Autodesk Fusion 360 part; units mm, degrees
(part 2 of 6)
  line L301 (104.1498, 9.6625) -> (103.164, 16.625)
  line L302 (105.0914, 15.125) -> (104.879, 16.625)
  line L303 (110.8723, 16.625) -> (111.8583, 9.6615)
  line L304 (105.0974, 9.5752) -> (105.8357, 8.8126)
  line L305 (104.679, 16.625) -> (105.5728, 10.3124)
  line L306 (110.938, 9.5499) -> (110.1997, 10.3126)
  line L307 (110.2123, 10.5871) -> (109.3574, 16.625)
  line L308 (104.879, 16.625) -> (109.1574, 16.625)
  line L309 (110.1997, 10.3126) -> (105.8609, 10.3126)
  line L310 (109.3574, 16.625) -> (110.8723, 16.625)
  line L311 (105.5728, 10.3124) -> (104.8998, 9.6625)
  line L312 (122.0778, 15.125) -> (117.7994, 15.125)
  line L313 (117.387, 16.625) -> (115.872, 16.625)
  arc A45 (125.0045, 2.5) -> (125.4996, 3.0701) centre (125.0045, 3) ccw
  circle A46 centre (115.872, 3.375) radius 0.875
  line L314 (117.6362, 9.4625) -> (118.5322, 8.5369)
  line L315 (124.0803, 2.5) -> (125.5803, 2.5)
  line L316 (123.6659, 4) -> (119.3766, 4)
  line L317 (118.5689, 10.3126) -> (117.8054, 9.5752)
  line L318 (119.387, 2.5) -> (117.872, 2.5)
  line L319 (117.872, 2.5) -> (116.8862, 9.4625)
  line L320 (123.1846, 8.8263) -> (124.0803, 2.5)
  line L321 (123.8783, 2.5) -> (123.6659, 4)
  line L322 (122.8824, 8.8126) -> (123.646, 9.5499)
  line L323 (124.5663, 9.6615) -> (123.8163, 9.6615)
  line L324 (125.5803, 2.5) -> (124.5944, 9.4635)
  arc A47 (116.4478, 16.625) -> (115.9527, 16.0549) centre (116.4478, 16.125) ccw
  line L325 (119.589, 2.5) -> (123.8783, 2.5)
  line L326 (118.5322, 8.5369) -> (119.387, 2.5)
  line L327 (123.8444, 9.4635) -> (123.1846, 8.8263)
  line L328 (119.3766, 4) -> (119.589, 2.5)
  line L329 (118.5437, 8.8126) -> (122.8824, 8.8126)
  line L330 (123.8163, 9.6615) -> (122.9203, 10.5871)
  line L331 (116.8862, 9.4625) -> (117.6362, 9.4625)
  line L332 (124.5944, 9.4635) -> (123.8444, 9.4635)
  arc A48 (117.8111, 2.9299) -> (118.3062, 2.5) centre (118.3062, 3) ccw
  line L333 (117.6078, 9.6625) -> (116.8578, 9.6625)
  line L334 (121.8654, 16.625) -> (122.0778, 15.125)
  arc A49 (123.6412, 16.1951) -> (123.1461, 16.625) centre (123.1461, 16.125) ccw
  line L335 (116.8578, 9.6625) -> (115.872, 16.625)
  line L336 (117.7994, 15.125) -> (117.587, 16.625)
  line L337 (123.5803, 16.625) -> (124.5663, 9.6615)
  line L338 (117.8054, 9.5752) -> (118.5437, 8.8126)
  line L339 (117.387, 16.625) -> (118.2808, 10.3124)
  line L340 (123.646, 9.5499) -> (122.9077, 10.3126)
  line L341 (122.9203, 10.5871) -> (122.0654, 16.625)
  line L342 (117.587, 16.625) -> (121.8654, 16.625)
  line L343 (122.9077, 10.3126) -> (118.5689, 10.3126)
  line L344 (122.0654, 16.625) -> (123.5803, 16.625)
  line L345 (118.2808, 10.3124) -> (117.6078, 9.6625)
  line L346 (134.7858, 15.125) -> (130.5074, 15.125)
  line L347 (130.095, 16.625) -> (128.58, 16.625)
  arc A50 (137.7125, 2.5) -> (138.2076, 3.0701) centre (137.7125, 3) ccw
  circle A51 centre (128.58, 3.375) radius 0.875
  line L348 (130.3442, 9.4625) -> (131.2402, 8.5369)
  line L349 (136.7883, 2.5) -> (138.2883, 2.5)
  line L350 (136.3739, 4) -> (132.0846, 4)
  line L351 (131.2769, 10.3126) -> (130.5134, 9.5752)
  line L352 (132.095, 2.5) -> (130.58, 2.5)
  line L353 (130.58, 2.5) -> (129.5942, 9.4625)
  line L354 (135.8926, 8.8263) -> (136.7883, 2.5)
  line L355 (136.5863, 2.5) -> (136.3739, 4)
  line L356 (135.5904, 8.8126) -> (136.354, 9.5499)
  line L357 (137.2743, 9.6615) -> (136.5243, 9.6615)
  line L358 (138.2883, 2.5) -> (137.3024, 9.4635)
  arc A52 (129.1558, 16.625) -> (128.6607, 16.0549) centre (129.1558, 16.125) ccw
  line L359 (132.297, 2.5) -> (136.5863, 2.5)
  line L360 (131.2402, 8.5369) -> (132.095, 2.5)
  line L361 (136.5524, 9.4635) -> (135.8926, 8.8263)
  line L362 (132.0846, 4) -> (132.297, 2.5)
  line L363 (131.2517, 8.8126) -> (135.5904, 8.8126)
  line L364 (136.5243, 9.6615) -> (135.6283, 10.5871)
  line L365 (129.5942, 9.4625) -> (130.3442, 9.4625)
  line L366 (137.3024, 9.4635) -> (136.5524, 9.4635)
  arc A53 (130.5191, 2.9299) -> (131.0142, 2.5) centre (131.0142, 3) ccw
  line L367 (130.3158, 9.6625) -> (129.5658, 9.6625)
  line L368 (134.5734, 16.625) -> (134.7858, 15.125)
  arc A54 (136.3492, 16.1951) -> (135.8541, 16.625) centre (135.8541, 16.125) ccw
  line L369 (129.5658, 9.6625) -> (128.58, 16.625)
  line L370 (130.5074, 15.125) -> (130.295, 16.625)
  line L371 (136.2883, 16.625) -> (137.2743, 9.6615)
  line L372 (130.5134, 9.5752) -> (131.2517, 8.8126)
  line L373 (130.095, 16.625) -> (130.9888, 10.3124)
  line L374 (136.354, 9.5499) -> (135.6157, 10.3126)
  line L375 (135.6283, 10.5871) -> (134.7734, 16.625)
  line L376 (130.295, 16.625) -> (134.5734, 16.625)
  line L377 (135.6157, 10.3126) -> (131.2769, 10.3126)
  line L378 (134.7734, 16.625) -> (136.2883, 16.625)
  line L379 (130.9888, 10.3124) -> (130.3158, 9.6625)
  line L380 (147.4938, 15.125) -> (143.2154, 15.125)
  line L381 (142.803, 16.625) -> (141.288, 16.625)
  arc A55 (150.4205, 2.5) -> (150.9156, 3.0701) centre (150.4205, 3) ccw
  circle A56 centre (141.288, 3.375) radius 0.875
  line L382 (143.0522, 9.4625) -> (143.9482, 8.5369)
  line L383 (149.4963, 2.5) -> (150.9963, 2.5)
  line L384 (149.0819, 4) -> (144.7926, 4)
  line L385 (143.9849, 10.3126) -> (143.2214, 9.5752)
  line L386 (144.803, 2.5) -> (143.288, 2.5)
  line L387 (143.288, 2.5) -> (142.3022, 9.4625)
  line L388 (148.6006, 8.8263) -> (149.4963, 2.5)
  line L389 (149.2943, 2.5) -> (149.0819, 4)
  line L390 (148.2984, 8.8126) -> (149.062, 9.5499)
  line L391 (149.9823, 9.6615) -> (149.2323, 9.6615)
  line L392 (150.9963, 2.5) -> (150.0104, 9.4635)
  arc A57 (141.8638, 16.625) -> (141.3687, 16.0549) centre (141.8638, 16.125) ccw
  line L393 (145.005, 2.5) -> (149.2943, 2.5)
  line L394 (143.9482, 8.5369) -> (144.803, 2.5)
  line L395 (149.2604, 9.4635) -> (148.6006, 8.8263)
  line L396 (144.7926, 4) -> (145.005, 2.5)
  line L397 (143.9597, 8.8126) -> (148.2984, 8.8126)
  line L398 (149.2323, 9.6615) -> (148.3363, 10.5871)
  line L399 (142.3022, 9.4625) -> (143.0522, 9.4625)
  line L400 (150.0104, 9.4635) -> (149.2604, 9.4635)
  arc A58 (143.2271, 2.9299) -> (143.7222, 2.5) centre (143.7222, 3) ccw
  line L401 (143.0238, 9.6625) -> (142.2738, 9.6625)
  line L402 (147.2814, 16.625) -> (147.4938, 15.125)
  arc A59 (149.0572, 16.1951) -> (148.5621, 16.625) centre (148.5621, 16.125) ccw
  line L403 (142.2738, 9.6625) -> (141.288, 16.625)
  line L404 (143.2154, 15.125) -> (143.003, 16.625)
  line L405 (148.9963, 16.625) -> (149.9823, 9.6615)
  line L406 (143.2214, 9.5752) -> (143.9597, 8.8126)
  line L407 (142.803, 16.625) -> (143.6968, 10.3124)
  line L408 (149.062, 9.5499) -> (148.3237, 10.3126)
  line L409 (148.3363, 10.5871) -> (147.4814, 16.625)
  line L410 (143.003, 16.625) -> (147.2814, 16.625)
  line L411 (148.3237, 10.3126) -> (143.9849, 10.3126)
  line L412 (147.4814, 16.625) -> (148.9963, 16.625)
  line L413 (143.6968, 10.3124) -> (143.0238, 9.6625)
  line L414 (160.2018, 15.125) -> (155.9234, 15.125)
  line L415 (155.511, 16.625) -> (153.996, 16.625)
  arc A60 (163.1285, 2.5) -> (163.6236, 3.0701) centre (163.1285, 3) ccw
  circle A61 centre (153.996, 3.375) radius 0.875
  line L416 (155.7602, 9.4625) -> (156.6562, 8.5369)
  line L417 (162.2043, 2.5) -> (163.7043, 2.5)
  line L418 (161.7899, 4) -> (157.5006, 4)
  line L419 (156.6929, 10.3126) -> (155.9294, 9.5752)
  line L420 (157.511, 2.5) -> (155.996, 2.5)
  line L421 (155.996, 2.5) -> (155.0102, 9.4625)
  line L422 (161.3086, 8.8263) -> (162.2043, 2.5)
  line L423 (162.0023, 2.5) -> (161.7899, 4)
  line L424 (161.0064, 8.8126) -> (161.77, 9.5499)
  line L425 (162.6903, 9.6615) -> (161.9403, 9.6615)
  line L426 (163.7043, 2.5) -> (162.7184, 9.4635)
  arc A62 (154.5718, 16.625) -> (154.0767, 16.0549) centre (154.5718, 16.125) ccw
  line L427 (157.713, 2.5) -> (162.0023, 2.5)
  line L428 (156.6562, 8.5369) -> (157.511, 2.5)
  line L429 (161.9684, 9.4635) -> (161.3086, 8.8263)
  line L430 (157.5006, 4) -> (157.713, 2.5)
  line L431 (156.6677, 8.8126) -> (161.0064, 8.8126)
  line L432 (161.9403, 9.6615) -> (161.0443, 10.5871)
  line L433 (155.0102, 9.4625) -> (155.7602, 9.4625)
  line L434 (162.7184, 9.4635) -> (161.9684, 9.4635)
  arc A63 (155.9351, 2.9299) -> (156.4302, 2.5) centre (156.4302, 3) ccw
  line L435 (155.7318, 9.6625) -> (154.9818, 9.6625)
  line L436 (159.9894, 16.625) -> (160.2018, 15.125)
  arc A64 (161.7652, 16.1951) -> (161.2701, 16.625) centre (161.2701, 16.125) ccw
  line L437 (154.9818, 9.6625) -> (153.996, 16.625)
  line L438 (155.9234, 15.125) -> (155.711, 16.625)
  line L439 (161.7043, 16.625) -> (162.6903, 9.6615)
  line L440 (155.9294, 9.5752) -> (156.6677, 8.8126)
  line L441 (155.511, 16.625) -> (156.4048, 10.3124)
  line L442 (161.77, 9.5499) -> (161.0317, 10.3126)
  line L443 (161.0443, 10.5871) -> (160.1894, 16.625)
  line L444 (155.711, 16.625) -> (159.9894, 16.625)
  line L445 (161.0317, 10.3126) -> (156.6929, 10.3126)
  line L446 (160.1894, 16.625) -> (161.7043, 16.625)
  line L447 (156.4048, 10.3124) -> (155.7318, 9.6625)
  line L448 (172.9098, 15.125) -> (168.6314, 15.125)
  line L449 (168.219, 16.625) -> (166.704, 16.625)
  arc A65 (175.8365, 2.5) -> (176.3316, 3.0701) centre (175.8365, 3) ccw
  circle A66 centre (166.704, 3.375) radius 0.875
  line L450 (168.4682, 9.4625) -> (169.3642, 8.5369)
  line L451 (174.9123, 2.5) -> (176.4123, 2.5)
  line L452 (174.4979, 4) -> (170.2086, 4)
  line L453 (169.4009, 10.3126) -> (168.6374, 9.5752)
  line L454 (170.219, 2.5) -> (168.704, 2.5)
  line L455 (168.704, 2.5) -> (167.7182, 9.4625)
  line L456 (174.0166, 8.8263) -> (174.9123, 2.5)
  line L457 (174.7103, 2.5) -> (174.4979, 4)
  line L458 (173.7144, 8.8126) -> (174.478, 9.5499)
  line L459 (175.3983, 9.6615) -> (174.6483, 9.6615)
  line L460 (176.4123, 2.5) -> (175.4264, 9.4635)
  arc A67 (167.2798, 16.625) -> (166.7847, 16.0549) centre (167.2798, 16.125) ccw
  line L461 (170.421, 2.5) -> (174.7103, 2.5)
  line L462 (169.3642, 8.5369) -> (170.219, 2.5)
  line L463 (174.6764, 9.4635) -> (174.0166, 8.8263)
  line L464 (170.2086, 4) -> (170.421, 2.5)
  line L465 (169.3757, 8.8126) -> (173.7144, 8.8126)
  line L466 (174.6483, 9.6615) -> (173.7523, 10.5871)
  line L467 (167.7182, 9.4625) -> (168.4682, 9.4625)
  line L468 (175.4264, 9.4635) -> (174.6764, 9.4635)
  arc A68 (168.6431, 2.9299) -> (169.1382, 2.5) centre (169.1382, 3) ccw
  line L469 (168.4398, 9.6625) -> (167.6898, 9.6625)
  line L470 (172.6974, 16.625) -> (172.9098, 15.125)
  arc A69 (174.4732, 16.1951) -> (173.9781, 16.625) centre (173.9781, 16.125) ccw
  line L471 (167.6898, 9.6625) -> (166.704, 16.625)
  line L472 (168.6314, 15.125) -> (168.419, 16.625)
  line L473 (174.4123, 16.625) -> (175.3983, 9.6615)
  line L474 (168.6374, 9.5752) -> (169.3757, 8.8126)
  line L475 (168.219, 16.625) -> (169.1128, 10.3124)
  line L476 (174.478, 9.5499) -> (173.7397, 10.3126)
  line L477 (173.7523, 10.5871) -> (172.8974, 16.625)
  line L478 (168.419, 16.625) -> (172.6974, 16.625)
  line L479 (173.7397, 10.3126) -> (169.4009, 10.3126)
  line L480 (172.8974, 16.625) -> (174.4123, 16.625)
  line L481 (169.1128, 10.3124) -> (168.4398, 9.6625)
  line L482 (185.6178, 15.125) -> (181.3394, 15.125)
  line L483 (180.927, 16.625) -> (179.412, 16.625)
  arc A70 (188.5445, 2.5) -> (189.0396, 3.0701) centre (188.5445, 3) ccw
  circle A71 centre (179.412, 3.375) radius 0.875
  line L484 (181.1762, 9.4625) -> (182.0722, 8.5369)
  line L485 (187.6203, 2.5) -> (189.1203, 2.5)
  line L486 (187.2059, 4) -> (182.9166, 4)
  line L487 (182.1089, 10.3126) -> (181.3454, 9.5752)
  line L488 (182.927, 2.5) -> (181.412, 2.5)
  line L489 (181.412, 2.5) -> (180.4262, 9.4625)
  line L490 (186.7246, 8.8263) -> (187.6203, 2.5)
  line L491 (187.4183, 2.5) -> (187.2059, 4)
  line L492 (186.4224, 8.8126) -> (187.186, 9.5499)
  line L493 (188.1063, 9.6615) -> (187.3563, 9.6615)
  line L494 (189.1203, 2.5) -> (188.1344, 9.4635)
  arc A72 (179.9878, 16.625) -> (179.4927, 16.0549) centre (179.9878, 16.125) ccw
  line L495 (183.129, 2.5) -> (187.4183, 2.5)
  line L496 (182.0722, 8.5369) -> (182.927, 2.5)
  line L497 (187.3844, 9.4635) -> (186.7246, 8.8263)
  line L498 (182.9166, 4) -> (183.129, 2.5)
  line L499 (182.0837, 8.8126) -> (186.4224, 8.8126)
  line L500 (187.3563, 9.6615) -> (186.4603, 10.5871)
  line L501 (180.4262, 9.4625) -> (181.1762, 9.4625)
  line L502 (188.1344, 9.4635) -> (187.3844, 9.4635)
  arc A73 (181.3511, 2.9299) -> (181.8462, 2.5) centre (181.8462, 3) ccw
  line L503 (181.1478, 9.6625) -> (180.3978, 9.6625)
  line L504 (185.4054, 16.625) -> (185.6178, 15.125)
  arc A74 (187.1812, 16.1951) -> (186.6861, 16.625) centre (186.6861, 16.125) ccw
  line L505 (180.3978, 9.6625) -> (179.412, 16.625)
  line L506 (181.3394, 15.125) -> (181.127, 16.625)
  line L507 (187.1203, 16.625) -> (188.1063, 9.6615)
  line L508 (181.3454, 9.5752) -> (182.0837, 8.8126)
  line L509 (180.927, 16.625) -> (181.8208, 10.3124)
  line L510 (187.186, 9.5499) -> (186.4477, 10.3126)
  line L511 (186.4603, 10.5871) -> (185.6054, 16.625)
  line L512 (181.127, 16.625) -> (185.4054, 16.625)
  line L513 (186.4477, 10.3126) -> (182.1089, 10.3126)
  line L514 (185.6054, 16.625) -> (187.1203, 16.625)
  line L515 (181.8208, 10.3124) -> (181.1478, 9.6625)
  line L516 (198.3258, 15.125) -> (194.0474, 15.125)
  line L517 (193.635, 16.625) -> (192.12, 16.625)
  arc A75 (201.2525, 2.5) -> (201.7476, 3.0701) centre (201.2525, 3) ccw
  circle A76 centre (192.12, 3.375) radius 0.875
  line L518 (193.8842, 9.4625) -> (194.7802, 8.5369)
  line L519 (200.3283, 2.5) -> (201.8283, 2.5)
  line L520 (199.9139, 4) -> (195.6246, 4)
  line L521 (194.8169, 10.3126) -> (194.0534, 9.5752)
  line L522 (195.635, 2.5) -> (194.12, 2.5)
  line L523 (194.12, 2.5) -> (193.1342, 9.4625)
  line L524 (199.4326, 8.8263) -> (200.3283, 2.5)
  line L525 (200.1263, 2.5) -> (199.9139, 4)
  line L526 (199.1304, 8.8126) -> (199.894, 9.5499)
  line L527 (200.8143, 9.6615) -> (200.0643, 9.6615)
  line L528 (201.8283, 2.5) -> (200.8424, 9.4635)
  arc A77 (192.6958, 16.625) -> (192.2007, 16.0549) centre (192.6958, 16.125) ccw
  line L529 (195.837, 2.5) -> (200.1263, 2.5)
  line L530 (194.7802, 8.5369) -> (195.635, 2.5)
  line L531 (200.0924, 9.4635) -> (199.4326, 8.8263)
  line L532 (195.6246, 4) -> (195.837, 2.5)
  line L533 (194.7917, 8.8126) -> (199.1304, 8.8126)
  line L534 (200.0643, 9.6615) -> (199.1683, 10.5871)
  line L535 (193.1342, 9.4625) -> (193.8842, 9.4625)
  line L536 (200.8424, 9.4635) -> (200.0924, 9.4635)
  arc A78 (194.0591, 2.9299) -> (194.5542, 2.5) centre (194.5542, 3) ccw
  line L537 (193.8558, 9.6625) -> (193.1058, 9.6625)
  line L538 (198.1134, 16.625) -> (198.3258, 15.125)
  arc A79 (199.8892, 16.1951) -> (199.3941, 16.625) centre (199.3941, 16.125) ccw
  line L539 (193.1058, 9.6625) -> (192.12, 16.625)
  line L540 (194.0474, 15.125) -> (193.835, 16.625)
  line L541 (199.8283, 16.625) -> (200.8143, 9.6615)
  line L542 (194.0534, 9.5752) -> (194.7917, 8.8126)
  line L543 (193.635, 16.625) -> (194.5288, 10.3124)
  line L544 (199.894, 9.5499) -> (199.1557, 10.3126)
  line L545 (199.1683, 10.5871) -> (198.3134, 16.625)
  line L546 (193.835, 16.625) -> (198.1134, 16.625)
  line L547 (199.1557, 10.3126) -> (194.8169, 10.3126)
  line L548 (198.3134, 16.625) -> (199.8283, 16.625)
  line L549 (194.5288, 10.3124) -> (193.8558, 9.6625)
  line L550 (7.7058, 34.25) -> (3.4274, 34.25)
  line L551 (3.015, 35.75) -> (1.5, 35.75)
  arc A80 (10.6325, 21.625) -> (11.1276, 22.1951) centre (10.6325, 22.125) ccw
  circle A81 centre (1.5, 22.5) radius 0.875
  line L552 (3.2642, 28.5875) -> (4.1602, 27.6619)
  line L553 (9.7083, 21.625) -> (11.2083, 21.625)
  line L554 (9.2939, 23.125) -> (5.0046, 23.125)
  line L555 (4.1969, 29.4376) -> (3.4334, 28.7002)
  line L556 (5.015, 21.625) -> (3.5, 21.625)
  line L557 (3.5, 21.625) -> (2.5142, 28.5875)
  line L558 (8.8126, 27.9513) -> (9.7083, 21.625)
  line L559 (9.5063, 21.625) -> (9.2939, 23.125)
  line L560 (8.5104, 27.9376) -> (9.274, 28.6749)
  line L561 (10.1943, 28.7865) -> (9.4443, 28.7865)
  line L562 (11.2083, 21.625) -> (10.2224, 28.5885)
  arc A82 (2.0758, 35.75) -> (1.5807, 35.1799) centre (2.0758, 35.25) ccw
  line L563 (5.217, 21.625) -> (9.5063, 21.625)
  line L564 (4.1602, 27.6619) -> (5.015, 21.625)
  line L565 (9.4724, 28.5885) -> (8.8126, 27.9513)
  line L566 (5.0046, 23.125) -> (5.217, 21.625)
  line L567 (4.1717, 27.9376) -> (8.5104, 27.9376)
  line L568 (9.4443, 28.7865) -> (8.5483, 29.7121)
  line L569 (2.5142, 28.5875) -> (3.2642, 28.5875)
  line L570 (10.2224, 28.5885) -> (9.4724, 28.5885)
  arc A83 (3.4391, 22.0549) -> (3.9342, 21.625) centre (3.9342, 22.125) ccw
  line L571 (3.2358, 28.7875) -> (2.4858, 28.7875)
  line L572 (7.4934, 35.75) -> (7.7058, 34.25)
  arc A84 (9.2692, 35.3201) -> (8.7741, 35.75) centre (8.7741, 35.25) ccw
  line L573 (2.4858, 28.7875) -> (1.5, 35.75)
  line L574 (3.4274, 34.25) -> (3.215, 35.75)
  line L575 (9.2083, 35.75) -> (10.1943, 28.7865)
  line L576 (3.4334, 28.7002) -> (4.1717, 27.9376)
  line L577 (3.015, 35.75) -> (3.9088, 29.4374)
  line L578 (9.274, 28.6749) -> (8.5357, 29.4376)
  line L579 (8.5483, 29.7121) -> (7.6934, 35.75)
  line L580 (3.215, 35.75) -> (7.4934, 35.75)
  line L581 (8.5357, 29.4376) -> (4.1969, 29.4376)
  line L582 (7.6934, 35.75) -> (9.2083, 35.75)
  line L583 (3.9088, 29.4374) -> (3.2358, 28.7875)
  line L584 (20.4138, 34.25) -> (16.1354, 34.25)
  line L585 (15.723, 35.75) -> (14.208, 35.75)
  arc A85 (23.3405, 21.625) -> (23.8356, 22.1951) centre (23.3405, 22.125) ccw
  circle A86 centre (14.208, 22.5) radius 0.875
  line L586 (15.9722, 28.5875) -> (16.8682, 27.6619)
  line L587 (22.4163, 21.625) -> (23.9163, 21.625)
  line L588 (22.0019, 23.125) -> (17.7126, 23.125)
  line L589 (16.9049, 29.4376) -> (16.1414, 28.7002)
  line L590 (17.723, 21.625) -> (16.208, 21.625)
  line L591 (16.208, 21.625) -> (15.2222, 28.5875)
  line L592 (21.5206, 27.9513) -> (22.4163, 21.625)
  line L593 (22.2143, 21.625) -> (22.0019, 23.125)
  line L594 (21.2184, 27.9376) -> (21.982, 28.6749)
  line L595 (22.9023, 28.7865) -> (22.1523, 28.7865)
  line L596 (23.9163, 21.625) -> (22.9304, 28.5885)
  arc A87 (14.7838, 35.75) -> (14.2887, 35.1799) centre (14.7838, 35.25) ccw
  line L597 (17.925, 21.625) -> (22.2143, 21.625)
  line L598 (16.8682, 27.6619) -> (17.723, 21.625)
  line L599 (22.1804, 28.5885) -> (21.5206, 27.9513)
  line L600 (17.7126, 23.125) -> (17.925, 21.625)
  line L601 (16.8797, 27.9376) -> (21.2184, 27.9376)
  line L602 (22.1523, 28.7865) -> (21.2563, 29.7121)
  line L603 (15.2222, 28.5875) -> (15.9722, 28.5875)
  line L604 (22.9304, 28.5885) -> (22.1804, 28.5885)
  arc A88 (16.1471, 22.0549) -> (16.6422, 21.625) centre (16.6422, 22.125) ccw
  line L605 (15.9438, 28.7875) -> (15.1938, 28.7875)
  line L606 (20.2014, 35.75) -> (20.4138, 34.25)
  arc A89 (21.9772, 35.3201) -> (21.4821, 35.75) centre (21.4821, 35.25) ccw
  line L607 (15.1938, 28.7875) -> (14.208, 35.75)
  line L608 (16.1354, 34.25) -> (15.923, 35.75)
  line L609 (21.9163, 35.75) -> (22.9023, 28.7865)
  line L610 (16.1414, 28.7002) -> (16.8797, 27.9376)
  line L611 (15.723, 35.75) -> (16.6168, 29.4374)
  line L612 (21.982, 28.6749) -> (21.2437, 29.4376)
  line L613 (21.2563, 29.7121) -> (20.4014, 35.75)
  line L614 (15.923, 35.75) -> (20.2014, 35.75)
  line L615 (21.2437, 29.4376) -> (16.9049, 29.4376)
  line L616 (20.4014, 35.75) -> (21.9163, 35.75)
  line L617 (16.6168, 29.4374) -> (15.9438, 28.7875)
  line L618 (33.1218, 34.25) -> (28.8434, 34.25)
  line L619 (28.431, 35.75) -> (26.916, 35.75)
  arc A90 (36.0485, 21.625) -> (36.5436, 22.1951) centre (36.0485, 22.125) ccw
  circle A91 centre (26.916, 22.5) radius 0.875
  line L620 (28.6802, 28.5875) -> (29.5762, 27.6619)
  line L621 (35.1243, 21.625) -> (36.6243, 21.625)
  line L622 (34.7099, 23.125) -> (30.4206, 23.125)
  line L623 (29.6129, 29.4376) -> (28.8494, 28.7002)
  line L624 (30.431, 21.625) -> (28.916, 21.625)
  line L625 (28.916, 21.625) -> (27.9302, 28.5875)
  line L626 (34.2286, 27.9513) -> (35.1243, 21.625)
  line L627 (34.9223, 21.625) -> (34.7099, 23.125)
  line L628 (33.9264, 27.9376) -> (34.69, 28.6749)
  line L629 (35.6103, 28.7865) -> (34.8603, 28.7865)
  line L630 (36.6243, 21.625) -> (35.6384, 28.5885)
  arc A92 (27.4918, 35.75) -> (26.9967, 35.1799) centre (27.4918, 35.25) ccw
  line L631 (30.633, 21.625) -> (34.9223, 21.625)
  line L632 (29.5762, 27.6619) -> (30.431, 21.625)
  line L633 (34.8884, 28.5885) -> (34.2286, 27.9513)
  line L634 (30.4206, 23.125) -> (30.633, 21.625)
  line L635 (29.5877, 27.9376) -> (33.9264, 27.9376)
  line L636 (34.8603, 28.7865) -> (33.9643, 29.7121)
  line L637 (27.9302, 28.5875) -> (28.6802, 28.5875)
  line L638 (35.6384, 28.5885) -> (34.8884, 28.5885)
  arc A93 (28.8551, 22.0549) -> (29.3502, 21.625) centre (29.3502, 22.125) ccw
  line L639 (28.6518, 28.7875) -> (27.9018, 28.7875)
  line L640 (32.9094, 35.75) -> (33.1218, 34.25)
  arc A94 (34.6852, 35.3201) -> (34.1901, 35.75) centre (34.1901, 35.25) ccw
  line L641 (27.9018, 28.7875) -> (26.916, 35.75)
  line L642 (28.8434, 34.25) -> (28.631, 35.75)
  line L643 (34.6243, 35.75) -> (35.6103, 28.7865)
  line L644 (28.8494, 28.7002) -> (29.5877, 27.9376)
  line L645 (28.431, 35.75) -> (29.3248, 29.4374)
  line L646 (34.69, 28.6749) -> (33.9517, 29.4376)
  line L647 (33.9643, 29.7121) -> (33.1094, 35.75)
  line L648 (28.631, 35.75) -> (32.9094, 35.75)
  line L649 (33.9517, 29.4376) -> (29.6129, 29.4376)
  line L650 (33.1094, 35.75) -> (34.6243, 35.75)
  line L651 (29.3248, 29.4374) -> (28.6518, 28.7875)
  line L652 (45.8298, 34.25) -> (41.5514, 34.25)
  line L653 (41.139, 35.75) -> (39.624, 35.75)
  arc A95 (48.7565, 21.625) -> (49.2516, 22.1951) centre (48.7565, 22.125) ccw
  circle A96 centre (39.624, 22.5) radius 0.875
  line L654 (41.3882, 28.5875) -> (42.2842, 27.6619)
  line L655 (47.8323, 21.625) -> (49.3323, 21.625)
  line L656 (47.4179, 23.125) -> (43.1286, 23.125)
  line L657 (42.3209, 29.4376) -> (41.5574, 28.7002)
  line L658 (43.139, 21.625) -> (41.624, 21.625)
  line L659 (41.624, 21.625) -> (40.6382, 28.5875)
  line L660 (46.9366, 27.9513) -> (47.8323, 21.625)
  line L661 (47.6303, 21.625) -> (47.4179, 23.125)
  line L662 (46.6344, 27.9376) -> (47.398, 28.6749)
  line L663 (48.3183, 28.7865) -> (47.5683, 28.7865)
  line L664 (49.3323, 21.625) -> (48.3464, 28.5885)
  arc A97 (40.1998, 35.75) -> (39.7047, 35.1799) centre (40.1998, 35.25) ccw
  line L665 (43.341, 21.625) -> (47.6303, 21.625)
  line L666 (42.2842, 27.6619) -> (43.139, 21.625)
  line L667 (47.5964, 28.5885) -> (46.9366, 27.9513)
  line L668 (43.1286, 23.125) -> (43.341, 21.625)
  line L669 (42.2957, 27.9376) -> (46.6344, 27.9376)
  line L670 (47.5683, 28.7865) -> (46.6723, 29.7121)
  line L671 (40.6382, 28.5875) -> (41.3882, 28.5875)
  line L672 (48.3464, 28.5885) -> (47.5964, 28.5885)
  arc A98 (41.5631, 22.0549) -> (42.0582, 21.625) centre (42.0582, 22.125) ccw
  line L673 (41.3598, 28.7875) -> (40.6098, 28.7875)
  line L674 (45.6174, 35.75) -> (45.8298, 34.25)
  arc A99 (47.3932, 35.3201) -> (46.8981, 35.75) centre (46.8981, 35.25) ccw
  line L675 (40.6098, 28.7875) -> (39.624, 35.75)
  line L676 (41.5514, 34.25) -> (41.339, 35.75)
  line L677 (47.3323, 35.75) -> (48.3183, 28.7865)
  line L678 (41.5574, 28.7002) -> (42.2957, 27.9376)
  line L679 (41.139, 35.75) -> (42.0328, 29.4374)
  line L680 (47.398, 28.6749) -> (46.6597, 29.4376)
  line L681 (46.6723, 29.7121) -> (45.8174, 35.75)
  line L682 (41.339, 35.75) -> (45.6174, 35.75)
  line L683 (46.6597, 29.4376) -> (42.3209, 29.4376)
  line L684 (45.8174, 35.75) -> (47.3323, 35.75)
  line L685 (42.0328, 29.4374) -> (41.3598, 28.7875)
  line L686 (58.5378, 34.25) -> (54.2594, 34.25)
  line L687 (53.847, 35.75) -> (52.332, 35.75)
  arc A100 (61.4645, 21.625) -> (61.9596, 22.1951) centre (61.4645, 22.125) ccw
  circle A101 centre (52.332, 22.5) radius 0.875
  line L688 (54.0962, 28.5875) -> (54.9922, 27.6619)
  line L689 (60.5403, 21.625) -> (62.0403, 21.625)
  line L690 (60.1259, 23.125) -> (55.8366, 23.125)
  line L691 (55.0289, 29.4376) -> (54.2654, 28.7002)
  line L692 (55.847, 21.625) -> (54.332, 21.625)
  line L693 (54.332, 21.625) -> (53.3462, 28.5875)
  line L694 (59.6446, 27.9513) -> (60.5403, 21.625)
  line L695 (60.3383, 21.625) -> (60.1259, 23.125)
  line L696 (59.3424, 27.9376) -> (60.106, 28.6749)
  line L697 (61.0263, 28.7865) -> (60.2763, 28.7865)
  line L698 (62.0403, 21.625) -> (61.0544, 28.5885)
  arc A102 (52.9078, 35.75) -> (52.4127, 35.1799) centre (52.9078, 35.25) ccw
  line L699 (56.049, 21.625) -> (60.3383, 21.625)
  line L700 (54.9922, 27.6619) -> (55.847, 21.625)
  line L701 (60.3044, 28.5885) -> (59.6446, 27.9513)
  line L702 (55.8366, 23.125) -> (56.049, 21.625)
  line L703 (55.0037, 27.9376) -> (59.3424, 27.9376)
  line L704 (60.2763, 28.7865) -> (59.3803, 29.7121)
  line L705 (53.3462, 28.5875) -> (54.0962, 28.5875)
  line L706 (61.0544, 28.5885) -> (60.3044, 28.5885)
  arc A103 (54.2711, 22.0549) -> (54.7662, 21.625) centre (54.7662, 22.125) ccw
  line L707 (54.0678, 28.7875) -> (53.3178, 28.7875)
  line L708 (58.3254, 35.75) -> (58.5378, 34.25)
  arc A104 (60.1012, 35.3201) -> (59.6061, 35.75) centre (59.6061, 35.25) ccw
  line L709 (53.3178, 28.7875) -> (52.332, 35.75)
  line L710 (54.2594, 34.25) -> (54.047, 35.75)
  line L711 (60.0403, 35.75) -> (61.0263, 28.7865)
  line L712 (54.2654, 28.7002) -> (55.0037, 27.9376)
  line L713 (53.847, 35.75) -> (54.7408, 29.4374)
  line L714 (60.106, 28.6749) -> (59.3677, 29.4376)
  line L715 (59.3803, 29.7121) -> (58.5254, 35.75)
  line L716 (54.047, 35.75) -> (58.3254, 35.75)
  line L717 (59.3677, 29.4376) -> (55.0289, 29.4376)
  line L718 (58.5254, 35.75) -> (60.0403, 35.75)
  line L719 (54.7408, 29.4374) -> (54.0678, 28.7875)
  line L720 (71.2458, 34.25) -> (66.9674, 34.25)
  line L721 (66.555, 35.75) -> (65.04, 35.75)
  arc A105 (74.1725, 21.625) -> (74.6676, 22.1951) centre (74.1725, 22.125) ccw
  circle A106 centre (65.04, 22.5) radius 0.875
  line L722 (66.8042, 28.5875) -> (67.7002, 27.6619)
  line L723 (73.2483, 21.625) -> (74.7483, 21.625)
  line L724 (72.8339, 23.125) -> (68.5446, 23.125)
  line L725 (67.7369, 29.4376) -> (66.9734, 28.7002)
  line L726 (68.555, 21.625) -> (67.04, 21.625)
  line L727 (67.04, 21.625) -> (66.0542, 28.5875)
  line L728 (72.3526, 27.9513) -> (73.2483, 21.625)
  line L729 (73.0463, 21.625) -> (72.8339, 23.125)
  line L730 (72.0504, 27.9376) -> (72.814, 28.6749)
  line L731 (73.7343, 28.7865) -> (72.9843, 28.7865)
  line L732 (74.7483, 21.625) -> (73.7624, 28.5885)
  arc A107 (65.6158, 35.75) -> (65.1207, 35.1799) centre (65.6158, 35.25) ccw
  line L733 (68.757, 21.625) -> (73.0463, 21.625)
  line L734 (67.7002, 27.6619) -> (68.555, 21.625)
  line L735 (73.0124, 28.5885) -> (72.3526, 27.9513)
  line L736 (68.5446, 23.125) -> (68.757, 21.625)
  line L737 (67.7117, 27.9376) -> (72.0504, 27.9376)
  line L738 (72.9843, 28.7865) -> (72.0883, 29.7121)
  line L739 (66.0542, 28.5875) -> (66.8042, 28.5875)
  line L740 (73.7624, 28.5885) -> (73.0124, 28.5885)
  arc A108 (66.9791, 22.0549) -> (67.4742, 21.625) centre (67.4742, 22.125) ccw
  line L741 (66.7758, 28.7875) -> (66.0258, 28.7875)
  line L742 (71.0334, 35.75) -> (71.2458, 34.25)
  arc A109 (72.8092, 35.3201) -> (72.3141, 35.75) centre (72.3141, 35.25) ccw
  line L743 (66.0258, 28.7875) -> (65.04, 35.75)
  line L744 (66.9674, 34.25) -> (66.755, 35.75)
  line L745 (72.7483, 35.75) -> (73.7343, 28.7865)
  line L746 (66.9734, 28.7002) -> (67.7117, 27.9376)
  line L747 (66.555, 35.75) -> (67.4488, 29.4374)
  line L748 (72.814, 28.6749) -> (72.0757, 29.4376)
  line L749 (72.0883, 29.7121) -> (71.2334, 35.75)
  line L750 (66.755, 35.75) -> (71.0334, 35.75)
  line L751 (72.0757, 29.4376) -> (67.7369, 29.4376)
  line L752 (71.2334, 35.75) -> (72.7483, 35.75)
  line L753 (67.4488, 29.4374) -> (66.7758, 28.7875)
  line L754 (83.9538, 34.25) -> (79.6754, 34.25)
  line L755 (79.263, 35.75) -> (77.748, 35.75)
  arc A110 (86.8805, 21.625) -> (87.3756, 22.1951) centre (86.8805, 22.125) ccw
  circle A111 centre (77.748, 22.5) radius 0.875
  line L756 (79.5122, 28.5875) -> (80.4082, 27.6619)
  line L757 (85.9563, 21.625) -> (87.4563, 21.625)
  line L758 (85.5419, 23.125) -> (81.2526, 23.125)
  line L759 (80.4449, 29.4376) -> (79.6814, 28.7002)
  line L760 (81.263, 21.625) -> (79.748, 21.625)
  line L761 (79.748, 21.625) -> (78.7622, 28.5875)
  line L762 (85.0606, 27.9513) -> (85.9563, 21.625)
  line L763 (85.7543, 21.625) -> (85.5419, 23.125)
  line L764 (84.7584, 27.9376) -> (85.522, 28.6749)
  line L765 (86.4423, 28.7865) -> (85.6923, 28.7865)
  line L766 (87.4563, 21.625) -> (86.4704, 28.5885)
  arc A112 (78.3238, 35.75) -> (77.8287, 35.1799) centre (78.3238, 35.25) ccw
  line L767 (81.465, 21.625) -> (85.7543, 21.625)
  line L768 (80.4082, 27.6619) -> (81.263, 21.625)
  line L769 (85.7204, 28.5885) -> (85.0606, 27.9513)
  line L770 (81.2526, 23.125) -> (81.465, 21.625)
  line L771 (80.4197, 27.9376) -> (84.7584, 27.9376)
  line L772 (85.6923, 28.7865) -> (84.7963, 29.7121)
  line L773 (78.7622, 28.5875) -> (79.5122, 28.5875)
  line L774 (86.4704, 28.5885) -> (85.7204, 28.5885)
  arc A113 (79.6871, 22.0549) -> (80.1822, 21.625) centre (80.1822, 22.125) ccw
  line L775 (79.4838, 28.7875) -> (78.7338, 28.7875)
  line L776 (83.7414, 35.75) -> (83.9538, 34.25)
  arc A114 (85.5172, 35.3201) -> (85.0221, 35.75) centre (85.0221, 35.25) ccw
  line L777 (78.7338, 28.7875) -> (77.748, 35.75)
  line L778 (79.6754, 34.25) -> (79.463, 35.75)
  line L779 (85.4563, 35.75) -> (86.4423, 28.7865)
  line L780 (79.6814, 28.7002) -> (80.4197, 27.9376)
  line L781 (79.263, 35.75) -> (80.1568, 29.4374)
  line L782 (85.522, 28.6749) -> (84.7837, 29.4376)
  line L783 (84.7963, 29.7121) -> (83.9414, 35.75)
  line L784 (79.463, 35.75) -> (83.7414, 35.75)
  line L785 (84.7837, 29.4376) -> (80.4449, 29.4376)
  line L786 (83.9414, 35.75) -> (85.4563, 35.75)
  line L787 (80.1568, 29.4374) -> (79.4838, 28.7875)
  line L788 (96.6618, 34.25) -> (92.3834, 34.25)
  line L789 (91.971, 35.75) -> (90.456, 35.75)
  arc A115 (99.5885, 21.625) -> (100.0836, 22.1951) centre (99.5885, 22.125) ccw
  circle A116 centre (90.456, 22.5) radius 0.875
  line L790 (92.2202, 28.5875) -> (93.1162, 27.6619)
  line L791 (98.6643, 21.625) -> (100.1643, 21.625)
  line L792 (98.2499, 23.125) -> (93.9606, 23.125)
  line L793 (93.1529, 29.4376) -> (92.3894, 28.7002)
  line L794 (93.971, 21.625) -> (92.456, 21.625)
  line L795 (92.456, 21.625) -> (91.4702, 28.5875)
  line L796 (97.7686, 27.9513) -> (98.6643, 21.625)
  line L797 (98.4623, 21.625) -> (98.2499, 23.125)
  line L798 (97.4664, 27.9376) -> (98.23, 28.6749)
  line L799 (99.1503, 28.7865) -> (98.4003, 28.7865)
  line L800 (100.1643, 21.625) -> (99.1784, 28.5885)
  arc A117 (91.0318, 35.75) -> (90.5367, 35.1799) centre (91.0318, 35.25) ccw
  line L801 (94.173, 21.625) -> (98.4623, 21.625)
  line L802 (93.1162, 27.6619) -> (93.971, 21.625)
  line L803 (98.4284, 28.5885) -> (97.7686, 27.9513)
  line L804 (93.9606, 23.125) -> (94.173, 21.625)
  line L805 (93.1277, 27.9376) -> (97.4664, 27.9376)
  line L806 (98.4003, 28.7865) -> (97.5043, 29.7121)
  line L807 (91.4702, 28.5875) -> (92.2202, 28.5875)
  line L808 (99.1784, 28.5885) -> (98.4284, 28.5885)
  arc A118 (92.3951, 22.0549) -> (92.8902, 21.625) centre (92.8902, 22.125) ccw
  line L809 (92.1918, 28.7875) -> (91.4418, 28.7875)
  line L810 (96.4494, 35.75) -> (96.6618, 34.25)
  arc A119 (98.2252, 35.3201) -> (97.7301, 35.75) centre (97.7301, 35.25) ccw
  line L811 (91.4418, 28.7875) -> (90.456, 35.75)
  line L812 (92.3834, 34.25) -> (92.171, 35.75)
  line L813 (98.1643, 35.75) -> (99.1503, 28.7865)
  line L814 (92.3894, 28.7002) -> (93.1277, 27.9376)
  line L815 (91.971, 35.75) -> (92.8648, 29.4374)
  line L816 (98.23, 28.6749) -> (97.4917, 29.4376)
  line L817 (97.5043, 29.7121) -> (96.6494, 35.75)
  line L818 (92.171, 35.75) -> (96.4494, 35.75)
  line L819 (97.4917, 29.4376) -> (93.1529, 29.4376)
  line L820 (96.6494, 35.75) -> (98.1643, 35.75)
  line L821 (92.8648, 29.4374) -> (92.1918, 28.7875)
  line L822 (109.3698, 34.25) -> (105.0914, 34.25)
  line L823 (104.679, 35.75) -> (103.164, 35.75)
  arc A120 (112.2965, 21.625) -> (112.7916, 22.1951) centre (112.2965, 22.125) ccw
  circle A121 centre (103.164, 22.5) radius 0.875
  line L824 (104.9282, 28.5875) -> (105.8242, 27.6619)
  line L825 (111.3723, 21.625) -> (112.8723, 21.625)
  line L826 (110.9579, 23.125) -> (106.6686, 23.125)
  line L827 (105.8609, 29.4376) -> (105.0974, 28.7002)
  line L828 (106.679, 21.625) -> (105.164, 21.625)
  line L829 (105.164, 21.625) -> (104.1782, 28.5875)
  line L830 (110.4766, 27.9513) -> (111.3723, 21.625)
  line L831 (111.1703, 21.625) -> (110.9579, 23.125)
  line L832 (110.1744, 27.9376) -> (110.938, 28.6749)
  line L833 (111.8583, 28.7865) -> (111.1083, 28.7865)
  line L834 (112.8723, 21.625) -> (111.8864, 28.5885)
  arc A122 (103.7398, 35.75) -> (103.2447, 35.1799) centre (103.7398, 35.25) ccw
  line L835 (106.881, 21.625) -> (111.1703, 21.625)
  line L836 (105.8242, 27.6619) -> (106.679, 21.625)
  line L837 (111.1364, 28.5885) -> (110.4766, 27.9513)
  line L838 (106.6686, 23.125) -> (106.881, 21.625)
  line L839 (105.8357, 27.9376) -> (110.1744, 27.9376)
  line L840 (111.1083, 28.7865) -> (110.2123, 29.7121)
  line L841 (104.1782, 28.5875) -> (104.9282, 28.5875)
  line L842 (111.8864, 28.5885) -> (111.1364, 28.5885)
  arc A123 (105.1031, 22.0549) -> (105.5982, 21.625) centre (105.5982, 22.125) ccw
  line L843 (104.8998, 28.7875) -> (104.1498, 28.7875)
  line L844 (109.1574, 35.75) -> (109.3698, 34.25)
  arc A124 (110.9332, 35.3201) -> (110.4381, 35.75) centre (110.4381, 35.25) ccw
  line L845 (104.1498, 28.7875) -> (103.164, 35.75)
  line L846 (105.0914, 34.25) -> (104.879, 35.75)
  line L847 (110.8723, 35.75) -> (111.8583, 28.7865)
  line L848 (105.0974, 28.7002) -> (105.8357, 27.9376)
  line L849 (104.679, 35.75) -> (105.5728, 29.4374)
  line L850 (110.938, 28.6749) -> (110.1997, 29.4376)
  line L851 (110.2123, 29.7121) -> (109.3574, 35.75)
  line L852 (104.879, 35.75) -> (109.1574, 35.75)
  line L853 (110.1997, 29.4376) -> (105.8609, 29.4376)
  line L854 (109.3574, 35.75) -> (110.8723, 35.75)
  line L855 (105.5728, 29.4374) -> (104.8998, 28.7875)
  line L856 (122.0778, 34.25) -> (117.7994, 34.25)
  line L857 (117.387, 35.75) -> (115.872, 35.75)
  arc A125 (125.0045, 21.625) -> (125.4996, 22.1951) centre (125.0045, 22.125) ccw
  circle A126 centre (115.872, 22.5) radius 0.875
  line L858 (117.6362, 28.5875) -> (118.5322, 27.6619)
  line L859 (124.0803, 21.625) -> (125.5803, 21.625)
  line L860 (123.6659, 23.125) -> (119.3766, 23.125)
  line L861 (118.5689, 29.4376) -> (117.8054, 28.7002)
  line L862 (119.387, 21.625) -> (117.872, 21.625)
  line L863 (117.872, 21.625) -> (116.8862, 28.5875)
  line L864 (123.1846, 27.9513) -> (124.0803, 21.625)
  line L865 (123.8783, 21.625) -> (123.6659, 23.125)
  line L866 (122.8824, 27.9376) -> (123.646, 28.6749)
  line L867 (124.5663, 28.7865) -> (123.8163, 28.7865)
  line L868 (125.5803, 21.625) -> (124.5944, 28.5885)
  arc A127 (116.4478, 35.75) -> (115.9527, 35.1799) centre (116.4478, 35.25) ccw
  line L869 (119.589, 21.625) -> (123.8783, 21.625)
  line L870 (118.5322, 27.6619) -> (119.387, 21.625)
  line L871 (123.8444, 28.5885) -> (123.1846, 27.9513)
  line L872 (119.3766, 23.125) -> (119.589, 21.625)
  line L873 (118.5437, 27.9376) -> (122.8824, 27.9376)
  line L874 (123.8163, 28.7865) -> (122.9203, 29.7121)
  line L875 (116.8862, 28.5875) -> (117.6362, 28.5875)
  line L876 (124.5944, 28.5885) -> (123.8444, 28.5885)
  arc A128 (117.8111, 22.0549) -> (118.3062, 21.625) centre (118.3062, 22.125) ccw
  line L877 (117.6078, 28.7875) -> (116.8578, 28.7875)
  line L878 (121.8654, 35.75) -> (122.0778, 34.25)
  arc A129 (123.6412, 35.3201) -> (123.1461, 35.75) centre (123.1461, 35.25) ccw
  line L879 (116.8578, 28.7875) -> (115.872, 35.75)
  line L880 (117.7994, 34.25) -> (117.587, 35.75)
  line L881 (123.5803, 35.75) -> (124.5663, 28.7865)
  line L882 (117.8054, 28.7002) -> (118.5437, 27.9376)
  line L883 (117.387, 35.75) -> (118.2808, 29.4374)
  line L884 (123.646, 28.6749) -> (122.9077, 29.4376)
  line L885 (122.9203, 29.7121) -> (122.0654, 35.75)
  line L886 (117.587, 35.75) -> (121.8654, 35.75)
  line L887 (122.9077, 29.4376) -> (118.5689, 29.4376)
  line L888 (122.0654, 35.75) -> (123.5803, 35.75)
  line L889 (118.2808, 29.4374) -> (117.6078, 28.7875)
  line L890 (134.7858, 34.25) -> (130.5074, 34.25)
  line L891 (130.095, 35.75) -> (128.58, 35.75)
  arc A130 (137.7125, 21.625) -> (138.2076, 22.1951) centre (137.7125, 22.125) ccw
  circle A131 centre (128.58, 22.5) radius 0.875
  line L892 (130.3442, 28.5875) -> (131.2402, 27.6619)
  line L893 (136.7883, 21.625) -> (138.2883, 21.625)
  line L894 (136.3739, 23.125) -> (132.0846, 23.125)
  line L895 (131.2769, 29.4376) -> (130.5134, 28.7002)
  line L896 (132.095, 21.625) -> (130.58, 21.625)
  line L897 (130.58, 21.625) -> (129.5942, 28.5875)
  line L898 (135.8926, 27.9513) -> (136.7883, 21.625)
  line L899 (136.5863, 21.625) -> (136.3739, 23.125)
  line L900 (135.5904, 27.9376) -> (136.354, 28.6749)
  line L901 (137.2743, 28.7865) -> (136.5243, 28.7865)
  line L902 (138.2883, 21.625) -> (137.3024, 28.5885)
  arc A132 (129.1558, 35.75) -> (128.6607, 35.1799) centre (129.1558, 35.25) ccw
  line L903 (132.297, 21.625) -> (136.5863, 21.625)
  line L904 (131.2402, 27.6619) -> (132.095, 21.625)
  line L905 (136.5524, 28.5885) -> (135.8926, 27.9513)
  line L906 (132.0846, 23.125) -> (132.297, 21.625)
  line L907 (131.2517, 27.9376) -> (135.5904, 27.9376)
  line L908 (136.5243, 28.7865) -> (135.6283, 29.7121)
  line L909 (129.5942, 28.5875) -> (130.3442, 28.5875)
  line L910 (137.3024, 28.5885) -> (136.5524, 28.5885)
  arc A133 (130.5191, 22.0549) -> (131.0142, 21.625) centre (131.0142, 22.125) ccw
  line L911 (130.3158, 28.7875) -> (129.5658, 28.7875)
  line L912 (134.5734, 35.75) -> (134.7858, 34.25)
  arc A134 (136.3492, 35.3201) -> (135.8541, 35.75) centre (135.8541, 35.25) ccw
  line L913 (129.5658, 28.7875) -> (128.58, 35.75)
  line L914 (130.5074, 34.25) -> (130.295, 35.75)
  line L915 (136.2883, 35.75) -> (137.2743, 28.7865)
  line L916 (130.5134, 28.7002) -> (131.2517, 27.9376)
  line L917 (130.095, 35.75) -> (130.9888, 29.4374)
  line L918 (136.354, 28.6749) -> (135.6157, 29.4376)
  line L919 (135.6283, 29.7121) -> (134.7734, 35.75)
  line L920 (130.295, 35.75) -> (134.5734, 35.75)
  line L921 (135.6157, 29.4376) -> (131.2769, 29.4376)
  line L922 (134.7734, 35.75) -> (136.2883, 35.75)
  line L923 (130.9888, 29.4374) -> (130.3158, 28.7875)
  line L924 (147.4938, 34.25) -> (143.2154, 34.25)
  line L925 (142.803, 35.75) -> (141.288, 35.75)
  arc A135 (150.4205, 21.625) -> (150.9156, 22.1951) centre (150.4205, 22.125) ccw
  circle A136 centre (141.288, 22.5) radius 0.875
  line L926 (143.0522, 28.5875) -> (143.9482, 27.6619)
  line L927 (149.4963, 21.625) -> (150.9963, 21.625)
  line L928 (149.0819, 23.125) -> (144.7926, 23.125)
  line L929 (143.9849, 29.4376) -> (143.2214, 28.7002)
  line L930 (144.803, 21.625) -> (143.288, 21.625)
  line L931 (143.288, 21.625) -> (142.3022, 28.5875)
  line L932 (148.6006, 27.9513) -> (149.4963, 21.625)
  line L933 (149.2943, 21.625) -> (149.0819, 23.125)
  line L934 (148.2984, 27.9376) -> (149.062, 28.6749)
  line L935 (149.9823, 28.7865) -> (149.2323, 28.7865)
  line L936 (150.9963, 21.625) -> (150.0104, 28.5885)
  arc A137 (141.8638, 35.75) -> (141.3687, 35.1799) centre (141.8638, 35.25) ccw
  line L937 (145.005, 21.625) -> (149.2943, 21.625)
  line L938 (143.9482, 27.6619) -> (144.803, 21.625)
  line L939 (149.2604, 28.5885) -> (148.6006, 27.9513)
  line L940 (144.7926, 23.125) -> (145.005, 21.625)
  line L941 (143.9597, 27.9376) -> (148.2984, 27.9376)
  line L942 (149.2323, 28.7865) -> (148.3363, 29.7121)
  line L943 (142.3022, 28.5875) -> (143.0522, 28.5875)
  line L944 (150.0104, 28.5885) -> (149.2604, 28.5885)
  arc A138 (143.2271, 22.0549) -> (143.7222, 21.625) centre (143.7222, 22.125) ccw
  line L945 (143.0238, 28.7875) -> (142.2738, 28.7875)
  line L946 (147.2814, 35.75) -> (147.4938, 34.25)
  arc A139 (149.0572, 35.3201) -> (148.5621, 35.75) centre (148.5621, 35.25) ccw
  line L947 (142.2738, 28.7875) -> (141.288, 35.75)
  line L948 (143.2154, 34.25) -> (143.003, 35.75)
  line L949 (148.9963, 35.75) -> (149.9823, 28.7865)
  line L950 (143.2214, 28.7002) -> (143.9597, 27.9376)
  line L951 (142.803, 35.75) -> (143.6968, 29.4374)
  line L952 (149.062, 28.6749) -> (148.3237, 29.4376)
  line L953 (148.3363, 29.7121) -> (147.4814, 35.75)
  line L954 (143.003, 35.75) -> (147.2814, 35.75)
  line L955 (148.3237, 29.4376) -> (143.9849, 29.4376)
  line L956 (147.4814, 35.75) -> (148.9963, 35.75)
  line L957 (143.6968, 29.4374) -> (143.0238, 28.7875)
  line L958 (160.2018, 34.25) -> (155.9234, 34.25)
  line L959 (155.511, 35.75) -> (153.996, 35.75)
  arc A140 (163.1285, 21.625) -> (163.6236, 22.1951) centre (163.1285, 22.125) ccw
  circle A141 centre (153.996, 22.5) radius 0.875
  line L960 (155.7602, 28.5875) -> (156.6562, 27.6619)
  line L961 (162.2043, 21.625) -> (163.7043, 21.625)
  line L962 (161.7899, 23.125) -> (157.5006, 23.125)
  line L963 (156.6929, 29.4376) -> (155.9294, 28.7002)
  line L964 (157.511, 21.625) -> (155.996, 21.625)
  line L965 (155.996, 21.625) -> (155.0102, 28.5875)
  line L966 (161.3086, 27.9513) -> (162.2043, 21.625)
  line L967 (162.0023, 21.625) -> (161.7899, 23.125)
  line L968 (161.0064, 27.9376) -> (161.77, 28.6749)
  line L969 (162.6903, 28.7865) -> (161.9403, 28.7865)
  line L970 (163.7043, 21.625) -> (162.7184, 28.5885)
  arc A142 (154.5718, 35.75) -> (154.0767, 35.1799) centre (154.5718, 35.25) ccw
  line L971 (157.713, 21.625) -> (162.0023, 21.625)
  line L972 (156.6562, 27.6619) -> (157.511, 21.625)
  line L973 (161.9684, 28.5885) -> (161.3086, 27.9513)
  line L974 (157.5006, 23.125) -> (157.713, 21.625)
  line L975 (156.6677, 27.9376) -> (161.0064, 27.9376)
  line L976 (161.9403, 28.7865) -> (161.0443, 29.7121)
  line L977 (155.0102, 28.5875) -> (155.7602, 28.5875)
  line L978 (162.7184, 28.5885) -> (161.9684, 28.5885)
  arc A143 (155.9351, 22.0549) -> (156.4302, 21.625) centre (156.4302, 22.125) ccw
  line L979 (155.7318, 28.7875) -> (154.9818, 28.7875)
  line L980 (159.9894, 35.75) -> (160.2018, 34.25)
  arc A144 (161.7652, 35.3201) -> (161.2701, 35.75) centre (161.2701, 35.25) ccw
  line L981 (154.9818, 28.7875) -> (153.996, 35.75)
  line L982 (155.9234, 34.25) -> (155.711, 35.75)
  line L983 (161.7043, 35.75) -> (162.6903, 28.7865)
  line L984 (155.9294, 28.7002) -> (156.6677, 27.9376)
  line L985 (155.511, 35.75) -> (156.4048, 29.4374)
  line L986 (161.77, 28.6749) -> (161.0317, 29.4376)
  line L987 (161.0443, 29.7121) -> (160.1894, 35.75)
  line L988 (155.711, 35.75) -> (159.9894, 35.75)
  line L989 (161.0317, 29.4376) -> (156.6929, 29.4376)
  line L990 (160.1894, 35.75) -> (161.7043, 35.75)
  line L991 (156.4048, 29.4374) -> (155.7318, 28.7875)
  line L992 (172.9098, 34.25) -> (168.6314, 34.25)
  line L993 (168.219, 35.75) -> (166.704, 35.75)
  arc A145 (175.8365, 21.625) -> (176.3316, 22.1951) centre (175.8365, 22.125) ccw
  circle A146 centre (166.704, 22.5) radius 0.875
  line L994 (168.4682, 28.5875) -> (169.3642, 27.6619)
  line L995 (174.9123, 21.625) -> (176.4123, 21.625)
  line L996 (174.4979, 23.125) -> (170.2086, 23.125)
  line L997 (169.4009, 29.4376) -> (168.6374, 28.7002)
  line L998 (170.219, 21.625) -> (168.704, 21.625)
  line L999 (168.704, 21.625) -> (167.7182, 28.5875)
  line L1000 (174.0166, 27.9513) -> (174.9123, 21.625)
  line L1001 (174.7103, 21.625) -> (174.4979, 23.125)
  line L1002 (173.7144, 27.9376) -> (174.478, 28.6749)
  line L1003 (175.3983, 28.7865) -> (174.6483, 28.7865)
  line L1004 (176.4123, 21.625) -> (175.4264, 28.5885)
  arc A147 (167.2798, 35.75) -> (166.7847, 35.1799) centre (167.2798, 35.25) ccw
  line L1005 (170.421, 21.625) -> (174.7103, 21.625)
  line L1006 (169.3642, 27.6619) -> (170.219, 21.625)
  line L1007 (174.6764, 28.5885) -> (174.0166, 27.9513)
  line L1008 (170.2086, 23.125) -> (170.421, 21.625)
  line L1009 (169.3757, 27.9376) -> (173.7144, 27.9376)
  line L1010 (174.6483, 28.7865) -> (173.7523, 29.7121)
  line L1011 (167.7182, 28.5875) -> (168.4682, 28.5875)
  line L1012 (175.4264, 28.5885) -> (174.6764, 28.5885)
  arc A148 (168.6431, 22.0549) -> (169.1382, 21.625) centre (169.1382, 22.125) ccw
  line L1013 (168.4398, 28.7875) -> (167.6898, 28.7875)
  line L1014 (172.6974, 35.75) -> (172.9098, 34.25)
  arc A149 (174.4732, 35.3201) -> (173.9781, 35.75) centre (173.9781, 35.25) ccw
  line L1015 (167.6898, 28.7875) -> (166.704, 35.75)
  line L1016 (168.6314, 34.25) -> (168.419, 35.75)
  line L1017 (174.4123, 35.75) -> (175.3983, 28.7865)
  line L1018 (168.6374, 28.7002) -> (169.3757, 27.9376)
  line L1019 (168.219, 35.75) -> (169.1128, 29.4374)
  line L1020 (174.478, 28.6749) -> (173.7397, 29.4376)
  line L1021 (173.7523, 29.7121) -> (172.8974, 35.75)
  line L1022 (168.419, 35.75) -> (172.6974, 35.75)
  line L1023 (173.7397, 29.4376) -> (169.4009, 29.4376)
  line L1024 (172.8974, 35.75) -> (174.4123, 35.75)
  line L1025 (169.1128, 29.4374) -> (168.4398, 28.7875)
  line L1026 (185.6178, 34.25) -> (181.3394, 34.25)
  line L1027 (180.927, 35.75) -> (179.412, 35.75)
  arc A150 (188.5445, 21.625) -> (189.0396, 22.1951) centre (188.5445, 22.125) ccw
  circle A151 centre (179.412, 22.5) radius 0.875
  line L1028 (181.1762, 28.5875) -> (182.0722, 27.6619)
  line L1029 (187.6203, 21.625) -> (189.1203, 21.625)
  line L1030 (187.2059, 23.125) -> (182.9166, 23.125)
  line L1031 (182.1089, 29.4376) -> (181.3454, 28.7002)
  line L1032 (182.927, 21.625) -> (181.412, 21.625)
  line L1033 (181.412, 21.625) -> (180.4262, 28.5875)
  line L1034 (186.7246, 27.9513) -> (187.6203, 21.625)
  line L1035 (187.4183, 21.625) -> (187.2059, 23.125)
  line L1036 (186.4224, 27.9376) -> (187.186, 28.6749)
  line L1037 (188.1063, 28.7865) -> (187.3563, 28.7865)
  line L1038 (189.1203, 21.625) -> (188.1344, 28.5885)
  arc A152 (179.9878, 35.75) -> (179.4927, 35.1799) centre (179.9878, 35.25) ccw
  line L1039 (183.129, 21.625) -> (187.4183, 21.625)
  line L1040 (182.0722, 27.6619) -> (182.927, 21.625)
  line L1041 (187.3844, 28.5885) -> (186.7246, 27.9513)
  line L1042 (182.9166, 23.125) -> (183.129, 21.625)
  line L1043 (182.0837, 27.9376) -> (186.4224, 27.9376)
  line L1044 (187.3563, 28.7865) -> (186.4603, 29.7121)
  line L1045 (180.4262, 28.5875) -> (181.1762, 28.5875)
  line L1046 (188.1344, 28.5885) -> (187.3844, 28.5885)
  arc A153 (181.3511, 22.0549) -> (181.8462, 21.625) centre (181.8462, 22.125) ccw
  line L1047 (181.1478, 28.7875) -> (180.3978, 28.7875)
  line L1048 (185.4054, 35.75) -> (185.6178, 34.25)
  arc A154 (187.1812, 35.3201) -> (186.6861, 35.75) centre (186.6861, 35.25) ccw
  line L1049 (180.3978, 28.7875) -> (179.412, 35.75)
  line L1050 (181.3394, 34.25) -> (181.127, 35.75)
  line L1051 (187.1203, 35.75) -> (188.1063, 28.7865)
  line L1052 (181.3454, 28.7002) -> (182.0837, 27.9376)
  line L1053 (180.927, 35.75) -> (181.8208, 29.4374)
  line L1054 (187.186, 28.6749) -> (186.4477, 29.4376)
  line L1055 (186.4603, 29.7121) -> (185.6054, 35.75)
  line L1056 (181.127, 35.75) -> (185.4054, 35.75)
  line L1057 (186.4477, 29.4376) -> (182.1089, 29.4376)
  line L1058 (185.6054, 35.75) -> (187.1203, 35.75)
  line L1059 (181.8208, 29.4374) -> (181.1478, 28.7875)
  line L1060 (198.3258, 34.25) -> (194.0474, 34.25)
  line L1061 (193.635, 35.75) -> (192.12, 35.75)
  arc A155 (201.2525, 21.625) -> (201.7476, 22.1951) centre (201.2525, 22.125) ccw
  circle A156 centre (192.12, 22.5) radius 0.875
  line L1062 (193.8842, 28.5875) -> (194.7802, 27.6619)
  line L1063 (200.3283, 21.625) -> (201.8283, 21.625)
  line L1064 (199.9139, 23.125) -> (195.6246, 23.125)
  line L1065 (194.8169, 29.4376) -> (194.0534, 28.7002)
  line L1066 (195.635, 21.625) -> (194.12, 21.625)
  line L1067 (194.12, 21.625) -> (193.1342, 28.5875)
  line L1068 (199.4326, 27.9513) -> (200.3283, 21.625)
  line L1069 (200.1263, 21.625) -> (199.9139, 23.125)
  line L1070 (199.1304, 27.9376) -> (199.894, 28.6749)
  line L1071 (200.8143, 28.7865) -> (200.0643, 28.7865)
  line L1072 (201.8283, 21.625) -> (200.8424, 28.5885)
  arc A157 (192.6958, 35.75) -> (192.2007, 35.1799) centre (192.6958, 35.25) ccw
  line L1073 (195.837, 21.625) -> (200.1263, 21.625)
  line L1074 (194.7802, 27.6619) -> (195.635, 21.625)
  line L1075 (200.0924, 28.5885) -> (199.4326, 27.9513)
  line L1076 (195.6246, 23.125) -> (195.837, 21.625)
  line L1077 (194.7917, 27.9376) -> (199.1304, 27.9376)
  line L1078 (200.0643, 28.7865) -> (199.1683, 29.7121)
  line L1079 (193.1342, 28.5875) -> (193.8842, 28.5875)
  line L1080 (200.8424, 28.5885) -> (200.0924, 28.5885)
  arc A158 (194.0591, 22.0549) -> (194.5542, 21.625) centre (194.5542, 22.125) ccw
  line L1081 (193.8558, 28.7875) -> (193.1058, 28.7875)
  line L1082 (198.1134, 35.75) -> (198.3258, 34.25)
  arc A159 (199.8892, 35.3201) -> (199.3941, 35.75) centre (199.3941, 35.25) ccw
  line L1083 (193.1058, 28.7875) -> (192.12, 35.75)
  line L1084 (194.0474, 34.25) -> (193.835, 35.75)
  line L1085 (199.8283, 35.75) -> (200.8143, 28.7865)
  line L1086 (194.0534, 28.7002) -> (194.7917, 27.9376)
  line L1087 (193.635, 35.75) -> (194.5288, 29.4374)
  line L1088 (199.894, 28.6749) -> (199.1557, 29.4376)
  line L1089 (199.1683, 29.7121) -> (198.3134, 35.75)
  line L1090 (193.835, 35.75) -> (198.1134, 35.75)
  line L1091 (199.1557, 29.4376) -> (194.8169, 29.4376)
  line L1092 (198.3134, 35.75) -> (199.8283, 35.75)
  line L1093 (194.5288, 29.4374) -> (193.8558, 28.7875)
  line L1094 (7.7058, 53.375) -> (3.4274, 53.375)
  line L1095 (3.015, 54.875) -> (1.5, 54.875)
  arc A160 (10.6325, 40.75) -> (11.1276, 41.3201) centre (10.6325, 41.25) ccw
  circle A161 centre (1.5, 41.625) radius 0.875
  line L1096 (3.2642, 47.7125) -> (4.1602, 46.7869)
  line L1097 (9.7083, 40.75) -> (11.2083, 40.75)